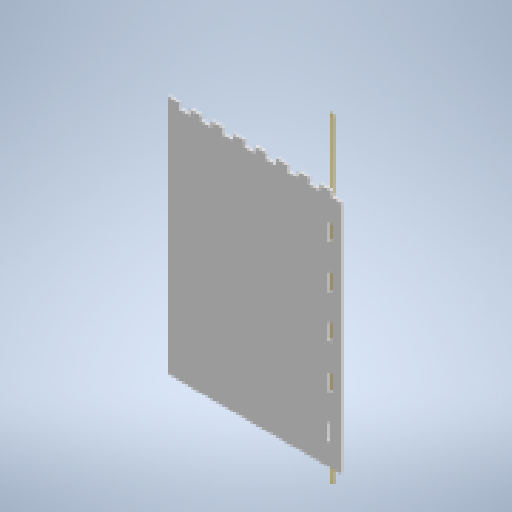
# Autodesk Inventor part: right back
Saved by Autodesk Inventor 2023 (Build 270158000, 158)
## iProperties
Created: 2023-09-18
Part Number: right back
Material: Polystyrene
Document SubType Name: Modeling
Designer: Nate
Mass: 679.87 g
Surface Area: 2892.38 cm^2
Volume: 665.887 cm^3
Density: 1.021 g/cm^3
Appearance: Smooth - White
Author: Nate
Autodesk Inventor part; units mm, degrees
ref_plane "YZ Plane" through (0, 0, 0) normal (1, 0, 0) x (0, 1, 0)
ref_plane "XZ Plane" through (0, 0, 0) normal (0, 1, 0) x (-1, 0, 0)
ref_plane "XY Plane" through (0, 0, 0) normal (0, 0, 1) x (1, 0, 0)
ref_plane "Work Plane1" through (0, 0, 0) normal (0, 0, 1) x (1, 0, 0)
sketch "Sketch1" plane through (0, 0, 0) normal (0, 0, 1) x (1, 0, 0)
  line L0 (0, 0) -> (-300, 0)
  line L1 (-300, 0) -> (-300, 434.166)
  line L2 (-300, 434.166) -> (0, 434.166)
  line L3 (0, 434.166) -> (0, 0)
  line L4 (0, 0) -> (20, 0)
  line L5 (20, 0) -> (20, 434.166)
  line L6 (20, 434.166) -> (0, 434.166)
  line L7 (0, 434.166) -> (0, 0)
  line L8 (0, 434.166) -> (-20, 434.166)
  line L9 (-20, 434.166) -> (-20, 444.166)
  line L10 (-20, 444.166) -> (0, 444.166)
  line L11 (0, 444.166) -> (0, 434.166)
  line L12 (-20, 434.166) -> (-40, 434.166)
  line L13 (-40, 434.166) -> (-40, 444.166)
  line L14 (-40, 444.166) -> (-20, 444.166)
  line L15 (-20, 444.166) -> (-20, 434.166)
  line L16 (-40, 434.166) -> (-60, 434.166)
  line L17 (-60, 434.166) -> (-60, 444.166)
  line L18 (-60, 444.166) -> (-40, 444.166)
  line L19 (-40, 444.166) -> (-40, 434.166)
  line L20 (-60, 434.166) -> (-80, 434.166)
  line L21 (-80, 434.166) -> (-80, 444.166)
  line L22 (-80, 444.166) -> (-60, 444.166)
  line L23 (-60, 444.166) -> (-60, 434.166)
  line L24 (-80, 434.166) -> (-100, 434.166)
  line L25 (-100, 434.166) -> (-100, 444.166)
  line L26 (-100, 444.166) -> (-80, 444.166)
  line L27 (-80, 444.166) -> (-80, 434.166)
  line L28 (-100, 434.166) -> (-120, 434.166)
  line L29 (-120, 434.166) -> (-120, 444.166)
  line L30 (-120, 444.166) -> (-100, 444.166)
  line L31 (-100, 444.166) -> (-100, 434.166)
  line L32 (-120, 434.166) -> (-140, 434.166)
  line L33 (-140, 434.166) -> (-140, 444.166)
  line L34 (-140, 444.166) -> (-120, 444.166)
  line L35 (-120, 444.166) -> (-120, 434.166)
  line L36 (-140, 434.166) -> (-160, 434.166)
  line L37 (-160, 434.166) -> (-160, 444.166)
  line L38 (-160, 444.166) -> (-140, 444.166)
  line L39 (-140, 444.166) -> (-140, 434.166)
  line L40 (-160, 434.166) -> (-180, 434.166)
  line L41 (-180, 434.166) -> (-180, 444.166)
  line L42 (-180, 444.166) -> (-160, 444.166)
  line L43 (-160, 444.166) -> (-160, 434.166)
  line L44 (-180, 434.166) -> (-200, 434.166)
  line L45 (-200, 434.166) -> (-200, 444.166)
  line L46 (-200, 444.166) -> (-180, 444.166)
  line L47 (-180, 444.166) -> (-180, 434.166)
  line L48 (-200, 434.166) -> (-220, 434.166)
  line L49 (-220, 434.166) -> (-220, 444.166)
  line L50 (-220, 444.166) -> (-200, 444.166)
  line L51 (-200, 444.166) -> (-200, 434.166)
  line L52 (-220, 434.166) -> (-240, 434.166)
  line L53 (-240, 434.166) -> (-240, 444.166)
  line L54 (-240, 444.166) -> (-220, 444.166)
  line L55 (-220, 444.166) -> (-220, 434.166)
  line L56 (-240, 434.166) -> (-260, 434.166)
  line L57 (-260, 434.166) -> (-260, 444.166)
  line L58 (-260, 444.166) -> (-240, 444.166)
  line L59 (-240, 444.166) -> (-240, 434.166)
  line L60 (-260, 434.166) -> (-280, 434.166)
  line L61 (-280, 434.166) -> (-280, 444.166)
  line L62 (-280, 444.166) -> (-260, 444.166)
  line L63 (-260, 444.166) -> (-260, 434.166)
  line L64 (-280, 434.166) -> (-300, 434.166)
  line L65 (-300, 434.166) -> (-300, 444.166)
  line L66 (-300, 444.166) -> (-280, 444.166)
  line L67 (-280, 444.166) -> (-280, 434.166)
  line L68 (0, 391.166) -> (-4.7625, 391.166)
  line L69 (-4.7625, 391.166) -> (-4.7625, 361.166)
  line L70 (-4.7625, 361.166) -> (0, 361.166)
  line L71 (0, 361.166) -> (0, 391.166)
  line L72 (0, 311.166) -> (-4.7625, 311.166)
  line L73 (-4.7625, 311.166) -> (-4.7625, 281.166)
  line L74 (-4.7625, 281.166) -> (0, 281.166)
  line L75 (0, 281.166) -> (0, 311.166)
  line L76 (0, 231.166) -> (-4.7625, 231.166)
  line L77 (-4.7625, 231.166) -> (-4.7625, 201.166)
  line L78 (-4.7625, 201.166) -> (0, 201.166)
  line L79 (0, 201.166) -> (0, 231.166)
  line L80 (0, 151.166) -> (-4.7625, 151.166)
  line L81 (-4.7625, 151.166) -> (-4.7625, 121.166)
  line L82 (-4.7625, 121.166) -> (0, 121.166)
  line L83 (0, 121.166) -> (0, 151.166)
  line L84 (-1.222, 71.166) -> (-5.9845, 71.166)
  line L85 (-5.9845, 71.166) -> (-5.9845, 41.166)
  line L86 (-5.9845, 41.166) -> (-1.222, 41.166)
  line L87 (-1.222, 41.166) -> (-1.222, 71.166)
  point P0 (-210, 444.166)
  point P1 (-210, 434.166)
  point P2 (-190, 434.166)
  point P3 (0, 361.166)
  dimension "d0" = 300
  dimension "d1" = 434.166
  dimension "d2" = 20
  dimension "d3" = 20
  dimension "d4" = 10
  dimension "d5" = 20
  dimension "d6" = 10
  dimension "d7" = 20
  dimension "d8" = 10
  dimension "d9" = 20
  dimension "d10" = 20
  dimension "d11" = 20
  dimension "d12" = 20
  dimension "d13" = 20
  dimension "d14" = 20
  dimension "d15" = 20
  dimension "d16" = 20
  dimension "d17" = 20
  dimension "d18" = 20
  dimension "d19" = 20
  dimension "d20" = 20
  dimension "d21" = 10
  dimension "d22" = 10
  dimension "d23" = 10
  dimension "d24" = 10
  dimension "d25" = 10
  dimension "d26" = 10
  dimension "d27" = 10
  dimension "d28" = 10
  dimension "d29" = 4.7625
  dimension "d30" = 30
  dimension "d31" = 4.7625
  dimension "d32" = 30
  dimension "d33" = 4.7625
  dimension "d34" = 30
  dimension "d35" = 4.7625
  dimension "d36" = 30
  dimension "d37" = 4.7625
  dimension "d38" = 30
  dimension "d39" = 43
  dimension "d40" = 50
  dimension "d41" = 50
  dimension "d42" = 50
  dimension "d43" = 50
  constraints: 176 end point, 44 parallel, 22 horizontal, 22 perpendicular, 10 point on line, 3 midpoint, 2 collinear
  measures "d0" distance of L1.end L2.end
  measures "d1" distance of L0.end L1.end
  measures "d2" distance of L6.end L5.end
  measures "d3" distance of L9.end L10.end
  measures "d4" distance between parallel lines of L10 L8
  measures "d5" distance of L13.end L14.end
  measures "d6" distance between parallel lines of L14 L2
  measures "d7" distance of L17.end L18.end
  measures "d8" distance between parallel lines of L18 L16
  measures "d9" distance of L21.end L22.end
  measures "d10" distance of L25.end L26.end
  measures "d11" distance of L29.end L30.end
  measures "d12" distance of L33.end L34.end
  measures "d13" distance of L37.end L38.end
  measures "d14" distance of L41.end L42.end
  measures "d15" distance of L45.end L46.end
  measures "d16" distance of L49.end L50.end
  measures "d17" distance between parallel lines of L49 L53
  measures "d18" distance of L57.end L58.end
  measures "d19" distance of L61.end L62.end
  measures "d20" distance of L65.end L66.end
  measures "d21" distance between parallel lines of L66 L2
  measures "d22" distance between parallel lines of L62 L2
  measures "d23" distance between parallel lines of L58 L2
  measures "d24" distance between parallel lines of L54 L2
  measures "d25" distance of point (-210, 444.166) point (-210, 434.166)
  measures "d26" distance from line of L46 point (-190, 434.166)
  measures "d27" distance between parallel lines of L42 L2
  measures "d28" distance between parallel lines of L38 L36
  measures "d29" distance of L70.end L69.end
  measures "d30" distance of L69.end L68.end
  measures "d31" distance of L75.start L74.start
  measures "d32" distance of L74.start L73.start
  measures "d33" distance of L79.start L78.start
  measures "d34" distance of L78.start L77.start
  measures "d35" distance of L83.start L82.start
  measures "d36" distance of L82.start L81.start
  measures "d37" distance of L87.start L86.start
  measures "d38" distance of L86.start L85.start
  measures "d39" distance between parallel lines of L2 L68
  measures "d40" distance between parallel lines of L70 L72
  measures "d41" distance between parallel lines of L78 L80
  measures "d42" distance between parallel lines of L82 L84
  measures "d43" distance between parallel lines of L74 L76
extrude "Extrusion1" add sketch "Sketch1" along normal blind 4.7625 contours L0 L1 L2 L3 L68 L69 L70 L72 L73 L74 L76 L77 L78 L80 L81 L82 | L3 L6 L5 L4 | L65 L66 L61 L2 | L2 L9 L10 L11 | L57 L58 L53 L2 | L2 L17 L18 L13 | L49 L50 L45 L2 | L2 L25 L26 L21 | L41 L42 L37 L2 | L2 L33 L34 L29
body "Solid1"
